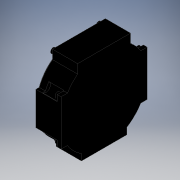
# Autodesk Inventor part: AKM2G-51DNCA_R
Saved by Autodesk Inventor 2019 (Build 230136000, 136)
## iProperties
Created: 2024-01-27
Part Number: AKM2G-51DNCA_R
Material: Generic
Catalog Web Link: www.cadenas.de
Description: AKM2G Size 5 - Rear-AKM2G Series
Vendor: KOLLMORGEN
Document SubType Name: Modeling
Designer: psAdmin
Manufacturer: KOLLMORGEN
Mass: 390.49 g
Surface Area: 388.694 cm^2
Volume: 390.49 cm^3
Density: 1 g/cm^3
Appearance: PSOLRGB-0-0-0
Category: PARTsolutions
Company: KOLLMORGEN
Title: AKM2G-51DNCA_R
Author: Cadenas PARTsolutions
Comments: AKM2G Series
PSOL_IDENT_0: {$CADENAS_DATA/23d-libs/kollmorgen/akm2g/parts/akm2g5_rear.prj},193 {VTYP=3D},{NB=AKM2G-51DNCA_R},{L
PSOL_IDENT_1: INA=AKM2G-51DNCA_R},{NN=AKM2G Size 5 - Rear},{DATE=19.05.2022 08:53:12},{GEOMDATE=01.03.2021 07:18:2
PSOL_IDENT_2: 6},{VERSION=},{LINEID=10},{WBVAR=CON,FD,BR,SL},{WBNUMERIC=}  {NB=AKM2G-51DNCA_R},{LINA=AKM2G-51DNCA_
PSOL_IDENT_3: R},{KT=DUMMY},{PN=AKM2G-51DNCA},{FS=Size 5},{CON=D},{FD=CA},{RL=29.4},{FDALG=  'CA', 'Sfd3 smart fee
PSOL_IDENT_4: dback', 'GU'  , 'Multi-turn hiperface dsl', 'LD', 'Multi-turn inductive endat 2.2'      },{BR=N},{L=
PSOL_IDENT_5: 141.9},{X=120.1},{SL=1},{A=57},{FDH=0},{M=21.1}
NB: AKM2G-51DNCA_R
NN: AKM2G Size 5 - Rear
NT: AKM2G Series
NBSYN: $PN._R
LINA: AKM2G-51DNCA_R
CATALOG: Kollmorgen
FS: Size 5
CON: Single right angle M23
FD: Sfd3 smart feedback
BR: No brake
SL: 1 Stack
M: 21.1
SUPPLIER: KOLLMORGEN
ARTICLENO: AKM2G-51DNCA_R
BOMINFO: AKM2G-51DNCA_R
CREATOR: CADENAS GmbH
Autodesk Inventor part; units mm, degrees
ref_plane "YZ Plane" through (0, 0, 0) normal (1, 0, 0) x (0, 1, 0)
ref_plane "XZ Plane" through (0, 0, 0) normal (0, 1, 0) x (-1, 0, 0)
ref_plane "XY Plane" through (0, 0, 0) normal (0, 0, 1) x (1, 0, 0)
sketch "Sketch_1" plane through (0, 0, 0) normal (1, 0, 0) x (0, 1, 0)
  line L0 (-22, 57) -> (-22, 52.5833)
  arc A0 (-22, 52.5833) -> (-48.4665, 30) centre (0, 0) ccw
  line L1 (-48.4665, 30) -> (-57, 30)
  line L2 (-57, 30) -> (-57, -30)
  line L3 (-57, -30) -> (-48.4665, -30)
  arc A1 (-48.4665, -30) -> (-22, -52.5833) centre (0, 0) ccw
  line L4 (-22, -52.5833) -> (-22, -57)
  line L5 (-22, -57) -> (22, -57)
  line L6 (22, -57) -> (22, -52.5833)
  arc A2 (22, -52.5833) -> (44.9889, -35) centre (0, 0) ccw
  line L7 (44.9889, -35) -> (57, -35)
  line L8 (57, -35) -> (57, 35)
  line L9 (57, 35) -> (44.9889, 35)
  arc A3 (44.9889, 35) -> (22, 52.5833) centre (0, 0) ccw
  line L10 (22, 52.5833) -> (22, 57)
  line L11 (22, 57) -> (-22, 57)
  constraints: 24 end point, 8 point on circle, 4 centre point
extrude "Extrusion1" add sketch "Sketch_1" along normal blind 29.4
sketch "Sketch_2" plane through (0, 0, 0) normal (1, 0, 0) x (0, 1, 0)
  line L0 (-17, 52) -> (-17, 49.1426)
  arc A0 (-17, 49.1426) -> (-49.1426, 17) centre (0, 0) ccw
  line L1 (-49.1426, 17) -> (-52, 17)
  line L2 (-52, 17) -> (-52, -17)
  line L3 (-52, -17) -> (-49.1426, -17)
  arc A1 (-49.1426, -17) -> (-17, -49.1426) centre (0, 0) ccw
  line L4 (-17, -49.1426) -> (-17, -52)
  line L5 (-17, -52) -> (17, -52)
  line L6 (17, -52) -> (17, -49.1426)
  arc A2 (17, -49.1426) -> (49.1426, -17) centre (0, 0) ccw
  line L7 (49.1426, -17) -> (52, -17)
  line L8 (52, -17) -> (52, 17)
  line L9 (52, 17) -> (49.1426, 17)
  arc A3 (49.1426, 17) -> (17, 49.1426) centre (0, 0) ccw
  line L10 (17, 49.1426) -> (17, 52)
  line L11 (17, 52) -> (-17, 52)
  constraints: 24 end point, 8 point on circle, 4 centre point
extrude "Extrusion2" add sketch "Sketch_2" against normal blind 7.9
sketch "Sketch_3" plane through (29.4, 0, 0) normal (1, 0, 0) x (0, 0, -1)
  line L0 (-57, 30) -> (-57, -30)
  line L1 (-57, -30) -> (57, -30)
  line L2 (57, -30) -> (57, 30)
  line L3 (57, 30) -> (-57, 30)
  constraints: 8 end point
extrude "Extrusion3" add sketch "Sketch_3" against normal blind 5
sketch "Sketch_7" plane through (0, 0, 0) normal (1, 0, 0) x (0, 1, 0)
  circle A0 centre (-52, -25) radius 3
  line L0 (-52.866, -23.5) -> (-53.7321, -25)
  line L1 (-53.7321, -25) -> (-52.866, -26.5)
  line L2 (-52.866, -26.5) -> (-51.134, -26.5)
  line L3 (-51.134, -26.5) -> (-50.2679, -25)
  line L4 (-50.2679, -25) -> (-51.134, -23.5)
  line L5 (-51.134, -23.5) -> (-52.866, -23.5)
  constraints: 12 end point, 1 centre point
extrude "Extrusion4" add sketch "Sketch_7" against normal blind 1
sketch "Sketch_8" plane through (24.4, 0, 0) normal (1, 0, 0) x (0, 0, -1)
  circle A0 centre (-52, 26) radius 6
  constraints: 1 centre point
extrude "Extrusion5" cut sketch "Sketch_8" against normal blind 20
sketch "Sketch_9" plane through (24.4, 0, 0) normal (1, 0, 0) x (0, 0, -1)
  circle A0 centre (52, 26) radius 6
  constraints: 1 centre point
extrude "Extrusion6" cut sketch "Sketch_9" against normal blind 20
sketch "Sketch_10" plane through (24.4, 0, 0) normal (1, 0, 0) x (0, 0, -1)
  circle A0 centre (-52, -26) radius 6
  constraints: 1 centre point
extrude "Extrusion7" cut sketch "Sketch_10" against normal blind 20
sketch "Sketch_11" plane through (24.4, 0, 0) normal (1, 0, 0) x (0, 0, -1)
  circle A0 centre (52, -26) radius 6
  constraints: 1 centre point
extrude "Extrusion8" cut sketch "Sketch_11" against normal blind 20
sketch "Sketch_12" plane through (24.4, 0, 0) normal (1, 0, 0) x (0, 0, -1)
  circle A0 centre (-53, 26) radius 3.5
  line L0 (-54.75, 24.9896) -> (-53, 23.9793)
  line L1 (-53, 23.9793) -> (-51.25, 24.9896)
  line L2 (-51.25, 24.9896) -> (-51.25, 27.0104)
  line L3 (-51.25, 27.0104) -> (-53, 28.0207)
  line L4 (-53, 28.0207) -> (-54.75, 27.0104)
  line L5 (-54.75, 27.0104) -> (-54.75, 24.9896)
  constraints: 12 end point, 1 centre point
extrude "Extrusion9" add sketch "Sketch_12" against normal blind 3.5
sketch "Sketch_13" plane through (24.4, 0, 0) normal (1, 0, 0) x (0, 0, -1)
  circle A0 centre (-53, -26) radius 3.5
  line L0 (-54.75, -27.0104) -> (-53, -28.0207)
  line L1 (-53, -28.0207) -> (-51.25, -27.0104)
  line L2 (-51.25, -27.0104) -> (-51.25, -24.9896)
  line L3 (-51.25, -24.9896) -> (-53, -23.9793)
  line L4 (-53, -23.9793) -> (-54.75, -24.9896)
  line L5 (-54.75, -24.9896) -> (-54.75, -27.0104)
  constraints: 12 end point, 1 centre point
extrude "Extrusion10" add sketch "Sketch_13" against normal blind 3.5
sketch "Sketch_14" plane through (24.4, 0, 0) normal (1, 0, 0) x (0, 0, -1)
  circle A0 centre (53, 26) radius 3.5
  line L0 (51.25, 24.9896) -> (53, 23.9793)
  line L1 (53, 23.9793) -> (54.75, 24.9896)
  line L2 (54.75, 24.9896) -> (54.75, 27.0104)
  line L3 (54.75, 27.0104) -> (53, 28.0207)
  line L4 (53, 28.0207) -> (51.25, 27.0104)
  line L5 (51.25, 27.0104) -> (51.25, 24.9896)
  constraints: 12 end point, 1 centre point
extrude "Extrusion11" add sketch "Sketch_14" against normal blind 3.5
sketch "Sketch_15" plane through (24.4, 0, 0) normal (1, 0, 0) x (0, 0, -1)
  circle A0 centre (53, -26) radius 3.5
  line L0 (51.25, -27.0104) -> (53, -28.0207)
  line L1 (53, -28.0207) -> (54.75, -27.0104)
  line L2 (54.75, -27.0104) -> (54.75, -24.9896)
  line L3 (54.75, -24.9896) -> (53, -23.9793)
  line L4 (53, -23.9793) -> (51.25, -24.9896)
  line L5 (51.25, -24.9896) -> (51.25, -27.0104)
  constraints: 12 end point, 1 centre point
extrude "Extrusion12" add sketch "Sketch_15" against normal blind 3.5
sketch "Sketch_21" plane through (0, 0, 0) normal (1, 0, 0) x (0, 1, 0)
  line L0 (-22, 57) -> (-22, 52.5833)
  arc A0 (-22, 52.5833) -> (-48.4665, 30) centre (0, 0) ccw
  line L1 (-48.4665, 30) -> (-57, 30)
  line L2 (-57, 30) -> (-57, -30)
  line L3 (-57, -30) -> (-48.4665, -30)
  arc A1 (-48.4665, -30) -> (-22, -52.5833) centre (0, 0) ccw
  line L4 (-22, -52.5833) -> (-22, -57)
  line L5 (-22, -57) -> (22, -57)
  line L6 (22, -57) -> (22, -52.5833)
  arc A2 (22, -52.5833) -> (44.9889, -35) centre (0, 0) ccw
  line L7 (44.9889, -35) -> (57, -35)
  line L8 (57, -35) -> (57, 35)
  line L9 (57, 35) -> (44.9889, 35)
  arc A3 (44.9889, 35) -> (22, 52.5833) centre (0, 0) ccw
  line L10 (22, 52.5833) -> (22, 57)
  line L11 (22, 57) -> (-22, 57)
  constraints: 24 end point, 8 point on circle, 4 centre point
extrude "Extrusion13" add sketch "Sketch_21" against normal blind 3.9
sketch "Sketch_22" plane through (-7.9, 0, 0) normal (1, 0, 0) x (0, 0, -1)
  circle A0 centre (30, 51) radius 3.5
  line L0 (28.25, 49.9896) -> (30, 48.9793)
  line L1 (30, 48.9793) -> (31.75, 49.9896)
  line L2 (31.75, 49.9896) -> (31.75, 52.0104)
  line L3 (31.75, 52.0104) -> (30, 53.0207)
  line L4 (30, 53.0207) -> (28.25, 52.0104)
  line L5 (28.25, 52.0104) -> (28.25, 49.9896)
  constraints: 12 end point, 1 centre point
extrude "Extrusion14" add sketch "Sketch_22" along normal blind 5
sketch "Sketch_4" plane through (-7.9, 0, 0) normal (1, 0, 0) x (0, 0, -1)
  circle A0 centre (-30, 51) radius 3.5
  line L0 (-31.75, 49.9896) -> (-30, 48.9793)
  line L1 (-30, 48.9793) -> (-28.25, 49.9896)
  line L2 (-28.25, 49.9896) -> (-28.25, 52.0104)
  line L3 (-28.25, 52.0104) -> (-30, 53.0207)
  line L4 (-30, 53.0207) -> (-31.75, 52.0104)
  line L5 (-31.75, 52.0104) -> (-31.75, 49.9896)
  constraints: 12 end point, 1 centre point
extrude "Extrusion15" add sketch "Sketch_4" along normal blind 5
sketch "Sketch_5" plane through (-7.9, 0, 0) normal (1, 0, 0) x (0, 0, -1)
  circle A0 centre (-25, -52) radius 3.5
  line L0 (-26.75, -53.0104) -> (-25, -54.0207)
  line L1 (-25, -54.0207) -> (-23.25, -53.0104)
  line L2 (-23.25, -53.0104) -> (-23.25, -50.9896)
  line L3 (-23.25, -50.9896) -> (-25, -49.9793)
  line L4 (-25, -49.9793) -> (-26.75, -50.9896)
  line L5 (-26.75, -50.9896) -> (-26.75, -53.0104)
  constraints: 12 end point, 1 centre point
extrude "Extrusion16" add sketch "Sketch_5" along normal blind 5
sketch "Sketch_6" plane through (-7.9, 0, 0) normal (1, 0, 0) x (0, 0, -1)
  circle A0 centre (25, -52) radius 3.5
  line L0 (23.25, -53.0104) -> (25, -54.0207)
  line L1 (25, -54.0207) -> (26.75, -53.0104)
  line L2 (26.75, -53.0104) -> (26.75, -50.9896)
  line L3 (26.75, -50.9896) -> (25, -49.9793)
  line L4 (25, -49.9793) -> (23.25, -50.9896)
  line L5 (23.25, -50.9896) -> (23.25, -53.0104)
  constraints: 12 end point, 1 centre point
extrude "Extrusion17" add sketch "Sketch_6" along normal blind 5
sketch "Sketch_24" plane through (-7.9, 0, 0) normal (-1, 0, 0) x (0, 0, 1)
  line L0 (-26.392, 13.3895) -> (-26.392, -13.3895)
  line L1 (-26.392, -13.3895) -> (26.392, -13.3895)
  line L2 (26.392, -13.3895) -> (26.392, 13.3895)
  line L3 (26.392, 13.3895) -> (-26.392, 13.3895)
  constraints: 8 end point
extrude "Extrusion18" cut sketch "Sketch_24" against normal blind 0.5
ref_plane "CON1_XY" through (14.8, 57, 16) normal (0, -1, 0) x (1, 0, 0)
ref_plane "CON1_YZ" through (14.8, 57, 16) normal (1, 0, 0) x (0, 0, 1)
ref_plane "CON1_ZX" through (14.8, 57, 16) normal (0, 0, 1) x (0, -1, 0)
ref_plane "CON2_XY" through (14.8, 57, -16) normal (0, -1, 0) x (1, 0, 0)
ref_plane "CON2_YZ" through (14.8, 57, -16) normal (1, 0, 0) x (0, 0, 1)
ref_plane "CON2_ZX" through (14.8, 57, -16) normal (0, 0, 1) x (0, -1, 0)
ref_plane "R_XY" through (29.4, 0, 0) normal (-1, 0, 0) x (0, 0, -1)
ref_plane "R_YZ" through (29.4, 0, 0) normal (0, 0, -1) x (0, -1, 0)
ref_plane "R_ZX" through (29.4, 0, 0) normal (0, -1, 0) x (-1, 0, 0)
body "Solid1"
